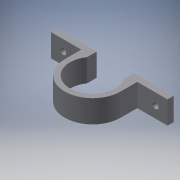
# Autodesk Inventor part: Rohrhalterung
Saved by Autodesk Inventor 2016 (Build 200138000, 138)
## iProperties
Created: 2015-06-23
Part Number: Rohrhalterung
Material: Generic
Document SubType Name: Modeling
Designer: Janine
Density: 1 g/cm^3
Appearance: Default
Author: Janine
Autodesk Inventor part; units mm, degrees
ref_plane "YZ Plane" through (0, 0, 0) normal (1, 0, 0) x (0, 1, 0)
ref_plane "XZ Plane" through (0, 0, 0) normal (0, 1, 0) x (-1, 0, 0)
ref_plane "XY Plane" through (0, 0, 0) normal (0, 0, 1) x (1, 0, 0)
sketch "Sketch1" plane through (0, 0, 0) normal (0, 1, 0) x (-1, 0, 0)
  arc A0 (12.2676, -8.6317) -> (-12.2676, -8.6317) centre (0, 0) ccw
  line L0 (-12.2676, -15) -> (-38.5, -15)
  arc A1 (18.5, 0) -> (-18.5, 0) centre (0, 0) ccw
  line L1 (-38.5, -15) -> (-38.5, -11)
  line L2 (-18.5, 0) -> (-18.5, -11)
  line L3 (-38.5, -11) -> (-18.5, -11)
  line L4 (-12.2676, -15) -> (-12.2676, -11)
  line L5 (-12.2676, -11) -> (-12.2676, -8.6317)
  line L6 (38.5, -11) -> (38.5, -15)
  line L7 (38.5, -15) -> (12.2676, -15)
  line L8 (18.5, 0) -> (18.5, -11)
  line L9 (18.5, -11) -> (38.5, -11)
  line L10 (12.2676, -8.6317) -> (12.2676, -15)
  dimension "d0" = 30
  dimension "d1" = 37
  dimension "d2" = 4
  dimension "d3" = 4
  dimension "d4" = 20
  dimension "d5" = 20
  constraints: 22 end point, 7 perpendicular, 4 point on circle, 3 tangent, 2 centre point, 2 coincident, 1 collinear, 1 horizontal
  measures "d0" diameter of A0
  measures "d1" diameter of A1
  measures "d2" distance of L0.end L1.end
  measures "d3" distance of L6.start L6.end
  measures "d4" distance of L1.end L2.end
  measures "d5" distance of L8.end L6.start
extrude "Extrusion1" add sketch "Sketch1" along normal blind 15
hole "Hole1" at (-30.5, 8, -11) direction (0, 0, -1) diameter 4 depth 8 tip angle 118
hole "Hole2" at (30.5, 7.5, -11) direction (0, 0, -1) diameter 4 depth 8 tip angle 118
body "Solid1"
